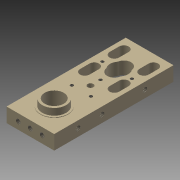
# Autodesk Inventor part: lower_part_01
Saved by Autodesk Inventor 2013 (Build 170138000, 138)
## iProperties
Created: 2014-01-07
Part Number: lower_part_01
Document SubType Name: Modeling
Designer: Ilja
Density: 1 g/cm^3
Material: Allgemein
Author: Ilja
Autodesk Inventor part; units mm, degrees
ref_plane "YZ Plane" through (0, 0, 0) normal (1, 0, 0) x (0, 1, 0)
ref_plane "XZ Plane" through (0, 0, 0) normal (0, 1, 0) x (-1, 0, 0)
ref_plane "XY Plane" through (0, 0, 0) normal (0, 0, 1) x (1, 0, 0)
sketch "Sketch1" plane through (0, 0, 0) normal (0, 0, 1) x (1, 0, 0)
  line L0 (0, 0) -> (50, 0)
  line L1 (50, 0) -> (50, 125)
  line L2 (50, 125) -> (0, 125)
  line L3 (0, 125) -> (0, 0)
  dimension "d0" = 50
  dimension "d1" = 125
  constraints: 8 end point, 2 parallel, 1 horizontal, 1 perpendicular
  measures "d0" distance of L0.start L0.end
  measures "d1" distance of L2.end L0.start
extrude "Extrusion1" add sketch "Sketch1" along normal blind 15
sketch "Sketch2" plane through (0, 0, 15) normal (0, 0, 1) x (1, 0, 0)
  point P0 (25, 25)
hole "Hole1" at (25, 25, 15) direction (0, 0, -1) diameter 20 end through all
sketch "Sketch3" plane through (0, 0, 15) normal (0, 0, 1) x (1, 0, 0)
  circle A0 centre (25, 25) radius 10 projected
  circle A1 centre (25, 25) radius 12.5
  dimension "d11" = 25
  constraints: 1 centre point, 1 coincident
  measures "d11" diameter of A1
extrude "Extrusion2" add sketch "Sketch3" along normal blind 7.5
sketch "Sketch4" plane through (0, 0, 0) normal (0, -1, 0) x (1, 0, 0)
  line L0 (50, 0) -> (50, 15) projected
  line L1 (50, 15) -> (0, 15) projected
  point P0 (12.5, 7.5)
  point P1 (25, 7.5)
  point P2 (37.5, 7.5)
  dimension "d14" = 12.5
  dimension "d15" = 12.5
  dimension "d16" = 12.5
  dimension "d152" = 7.5
  dimension "d153" = 7.5
  dimension "d154" = 7.5
  measures "d14" distance of point (25, 7.5) point (12.5, 7.5)
  measures "d15" distance of point (37.5, 7.5) point (25, 7.5)
  measures "d16" distance from line of L0 point (37.5, 7.5)
  measures "d152" distance from line of L1 point (12.5, 7.5)
  measures "d153" distance from line of L1 point (25, 7.5)
  measures "d154" distance from line of L1 point (37.5, 7.5)
hole "Hole2" at (12.5, 0, 7.5) at (25, 0, 7.5) at (37.5, 0, 7.5) direction (0, 1, 0) diameter 4.917 depth 10 tip angle 118 thread size "M6x1" class "6H" standard "ANSI Metric M Profile"
sketch "Sketch10" plane through (50, 0, 0) normal (1, 0, 0) x (0, 0, -1)
  line L0 (-15, 125) -> (-15, 0) projected
  line L1 (0, 0) -> (-15, 0) projected
  line L2 (0, 125) -> (-15, 125) projected
  point P0 (-7.5, 25)
  point P1 (-7.5, 50)
  point P2 (-7.5, 95)
  dimension "d112" = 7.5
  dimension "d113" = 25
  dimension "d114" = 25
  dimension "d118" = 30
  dimension "d150" = 7.5
  measures "d112" distance from line of point (-7.5, 25) L0
  measures "d113" distance from line of L1 point (-7.5, 25)
  measures "d114" distance of point (-7.5, 25) point (-7.5, 50)
  measures "d118" distance from line of L2 point (-7.5, 95)
  measures "d150" distance from line of L0 point (-7.5, 95)
hole "Hole8" at (50, 25, 7.5) at (50, 50, 7.5) at (50, 95, 7.5) direction (-1, 0, 0) diameter 4.917 depth 8 tip angle 118 thread size "M6x1" class "6H" standard "ANSI Metric M Profile"
sketch "Sketch11" plane through (0, 0, 0) normal (-1, 0, 0) x (0, 0, 1)
  circle A0 centre (7.5, 25) radius 2.4585 projected
  line L0 (0, 125) -> (15, 125) projected
  line L1 (0, 0) -> (15, 0) projected
  line L2 (15, 0) -> (15, 125) projected
  point P0 (7.5, 50)
  point P1 (7.5, 95)
  dimension "d119" = 25
  dimension "d120" = 25
  dimension "d121" = 30
  dimension "d151" = 7.5
  measures "d119" distance from line of L1 A0.centre
  measures "d120" distance of point (7.5, 50) A0.centre
  measures "d121" distance from line of L0 point (7.5, 95)
  measures "d151" distance from line of L2 point (7.5, 95)
hole "Hole9" at (0, 25, 7.5) at (0, 50, 7.5) at (0, 95, 7.5) direction (1, 0, 0) diameter 4.917 depth 8 tip angle 118 thread size "M6x1" class "6H" standard "ANSI Metric M Profile"
sketch "Skizze12" plane through (0, 0, 0) normal (0, 0, -1) x (-1, 0, 0)
  line L0 (-50, 0) -> (-50, 125) projected
  line L1 (-50, 125) -> (0, 125) projected
  arc A0 (-17.5, 98) -> (-32.5, 98) centre (-25, 98) ccw
  arc A1 (-32.5, 88) -> (-17.5, 88) centre (-25, 88) ccw
  line L2 (-32.5, 88) -> (-32.5, 98)
  line L3 (-17.5, 98) -> (-17.5, 88)
  arc A2 (-36.1, 88) -> (-13.9, 88) centre (-25, 88) ccw
  line L4 (-36.1, 88) -> (-36.1, 98)
  line L5 (-13.9, 98) -> (-13.9, 88)
  arc A3 (-13.9, 98) -> (-36.1, 98) centre (-25, 98) ccw
  point P0 (-45, 115)
  point P1 (-50, 110)
  point P2 (-5, 115)
  point P3 (0, 125)
  point P4 (-25, 93)
  dimension "d80" = 15
  dimension "d81" = 25
  dimension "d82" = 27
  dimension "d83" = 15
  dimension "d84" = 10
  dimension "d86" = 22.2
  constraints: 8 end point, 8 point on circle, 6 tangent, 4 centre point, 2 coincident, 1 other
  measures "d80" diameter of A0
  measures "d81" distance from line of L0 A0.centre
  measures "d83" diameter of A1
  measures "d84" distance of A0.centre A1.centre
  measures "d86" diameter of A2
extrude "Extrusion5" cut sketch "Skizze12" against normal blind 17 contours L3 A1 L2 A0
extrude "Extrusion6" cut sketch "Skizze12" against normal blind 2
sketch "Skizze13" plane through (0, 0, 15) normal (0, 0, 1) x (1, 0, 0)
  arc A0 (32.5, 98) -> (17.5, 98) centre (25, 98) ccw projected
  arc A1 (11.25, 113.5) -> (7.75, 113.5) centre (9.5, 113.5) ccw
  arc A2 (7.75, 103.5) -> (11.25, 103.5) centre (9.5, 103.5) ccw
  arc A3 (14.5, 113.5) -> (4.5, 113.5) centre (9.5, 113.5) ccw
  arc A4 (4.5, 103.5) -> (14.5, 103.5) centre (9.5, 103.5) ccw
  line L0 (4.5, 103.5) -> (4.5, 113.5)
  line L1 (14.5, 103.5) -> (14.5, 113.5)
  line L2 (7.75, 103.5) -> (7.75, 113.5)
  line L3 (11.25, 103.5) -> (11.25, 113.5)
  dimension "d95" = 3.5
  dimension "d96" = 3.5
  dimension "d97" = 10
  dimension "d98" = 15.5
  dimension "d99" = 10
  dimension "d100" = 10
  dimension "d111" = 15.5
  constraints: 8 end point, 8 point on circle, 8 tangent, 4 centre point, 2 coincident
  measures "d95" diameter of A1
  measures "d96" diameter of A2
  measures "d97" distance of A1.centre A2.centre
  measures "d98" horizontal distance of A0.centre A1.centre
  measures "d99" diameter of A3
  measures "d100" diameter of A4
  measures "d111" horizontal distance of A0.centre A1.centre
extrude "Extrusion7" cut sketch "Skizze13" against normal blind 17 contours L3 A2 L2 A1
extrude "Extrusion8" cut sketch "Skizze13" against normal blind 10
pattern_linear "Rechteckige Anordnung1" count 2 spacing 31 along (0, -1, 0) count 2 spacing 31 along (1, 0, 0) of "Extrusion8", "Extrusion7"
sketch "Skizze14" plane through (0, 125, 0) normal (0, 1, 0) x (1, 0, 0)
  line L0 (50, 0) -> (50, -15) projected
  line L1 (0, -15) -> (50, -15) projected
  point P0 (25, -7.5)
  dimension "d124" = 25
  dimension "d155" = 7.5
  measures "d124" distance from line of L0 point (25, -7.5)
  measures "d155" distance from line of L1 point (25, -7.5)
hole "Bohrung10" at (25, 125, 7.5) direction (0, -1, 0) diameter 4.917 depth 12 tip angle 118 thread size "M6x1" class "6H" standard "ANSI Metric M Profile"
sketch "Skizze15" plane through (0, 0, 15) normal (0, 0, 1) x (1, 0, 0)
  arc A0 (32.5, 98) -> (17.5, 98) centre (25, 98) ccw projected
  point P0 (9.5, 91)
  point P1 (40.5, 91)
  point P2 (25, 73.5)
  point P3 (35, 53.5)
  point P4 (15, 53.5)
  dimension "d132" = 17.5
  dimension "d133" = 17.5
  dimension "d134" = 7
  dimension "d159" = 20
  dimension "d160" = 10
  dimension "d161" = 10
  dimension "d162" = 20
  measures "d132" vertical distance of point (9.5, 91) point (25, 73.5)
  measures "d133" vertical distance of point (40.5, 91) point (25, 73.5)
  measures "d134" vertical distance of A0.centre point (9.5, 91)
  measures "d159" vertical distance of point (35, 53.5) point (25, 73.5)
  measures "d160" horizontal distance of point (35, 53.5) point (25, 73.5)
  measures "d161" horizontal distance of point (15, 53.5) point (25, 73.5)
  measures "d162" vertical distance of point (15, 53.5) point (25, 73.5)
hole "Bohrung11" at (9.5, 91, 15) at (40.5, 91, 15) at (25, 73.5, 15) at (35, 53.5, 15) at (15, 53.5, 15) direction (0, 0, -1) diameter 3.242 end through all thread size "M4x0.7" class "6H" standard "ANSI Metric M Profile"
sketch "Skizze16" plane through (0, 0, 15) normal (0, 0, 1) x (1, 0, 0)
  arc A0 (17.5, 88) -> (32.5, 88) centre (25, 88) ccw projected
  point P0 (25, 63)
  dimension "d142" = 25
  measures "d142" distance of A0.centre point (25, 63)
hole "Bohrung12" at (25, 63, 15) direction (0, 0, -1) diameter 6 end through all
sketch "Skizze17" plane through (0, 0, 15) normal (0, 0, 1) x (1, 0, 0)
  circle A0 centre (25, 25) radius 12.5 projected
  circle A1 centre (25, 25) radius 14.5
  dimension "d163" = 29
  constraints: 1 centre point, 1 coincident
  measures "d163" diameter of A1
extrude "Extrusion9" add sketch "Skizze17" along normal blind 0.5
hole "Bohrung13" at (25, 93, 0) direction (0, 0, 1) diameter 19 end through all
equation "\"d83\" = d80"
equation "\"d96\" = d95"
equation "\"d100\" = d99"
equation "\"d133\" = d132"
equation "\"d161\" = d160"
equation "\"d162\" = d159"
body "Solid1"
